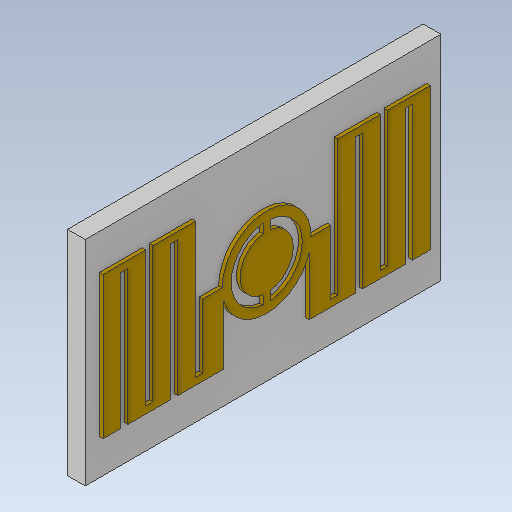
# Autodesk Inventor part: MEMS
Saved by Autodesk Inventor 2020 (Build 240168000, 168)
## iProperties
Created: 2018-12-01
Part Number: MEMS
Material: Generic
Document SubType Name: Modeling
Designer: Ralf
Density: 1 g/cm^3
Appearance: Default
Author: Ralf
Autodesk Inventor part; units mm, degrees
ref_plane "YZ Plane" through (0, 0, 0) normal (1, 0, 0) x (0, 1, 0)
ref_plane "XZ Plane" through (0, 0, 0) normal (0, 1, 0) x (-1, 0, 0)
ref_plane "XY Plane" through (0, 0, 0) normal (0, 0, 1) x (1, 0, 0)
sketch "Sketch1" plane through (0, 0, 0) normal (1, 0, 0) x (0, 1, 0)
  line L0 (-3, 5) -> (3, 5)
  line L1 (3, 5) -> (3, -5)
  line L2 (3, -5) -> (-3, -5)
  line L3 (-3, -5) -> (-3, 5)
  point P0 (0, 0)
  dimension "d0" = 6
  dimension "d1" = 10
  dimension "d2" = 3
  dimension "d3" = 5
  constraints: 8 end point, 2 parallel, 1 horizontal, 1 perpendicular
  measures "d0" distance of L0.start L0.end
  measures "d1" distance of L0.end L1.end
  measures "d2" distance from line of point (0, 0) L3
  measures "d3" distance from line of point (0, 0) L2
extrude "Extrusion1" add sketch "Sketch1" along normal blind 0.5
sketch "Sketch2" plane through (0.5, 0, 0) normal (1, 0, 0) x (0, 0, -1)
  circle A0 centre (0, 0) radius 0.75
  circle A1 centre (0, 0) radius 1
  circle A2 centre (0, 0) radius 1.25
  line L0 (-2.5, -2) -> (-2, -2)
  line L1 (-2, -2) -> (-2, 2)
  line L2 (-2, 2) -> (-2.5, 2)
  line L3 (-2.5, 2) -> (-2.5, -2)
  line L4 (-5, -3) -> (5, -3) projected
  line L5 (-3.2, -2) -> (-2.7, -2)
  line L6 (-2.7, -2) -> (-2.7, 2)
  line L7 (-2.7, 2) -> (-3.2, 2)
  line L8 (-3.2, 2) -> (-3.2, -2)
  line L9 (-3.9, -2) -> (-3.4, -2)
  line L10 (-3.4, -2) -> (-3.4, 2)
  line L11 (-3.4, 2) -> (-3.9, 2)
  line L12 (-3.9, 2) -> (-3.9, -2)
  line L13 (-4.6, -2) -> (-4.1, -2)
  line L14 (-4.1, -2) -> (-4.1, 2)
  line L15 (-4.1, 2) -> (-4.6, 2)
  line L16 (-4.6, 2) -> (-4.6, -2)
  line L17 (-0.1, -1.1173) -> (0.1, -1.1173)
  line L18 (0.1, -1.1173) -> (0.1, 1.1584)
  line L19 (0.1, 1.1584) -> (-0.1, 1.1584)
  line L20 (-0.1, 1.1584) -> (-0.1, -1.1173)
  line L21 (-1.8, -2) -> (-1.2, -2)
  line L22 (-1.2, -2) -> (-1.2, 0)
  line L23 (-1.2, 0) -> (-1.8, 0)
  line L24 (-1.8, 0) -> (-1.8, -2)
  line L25 (-1.8, -2) -> (-2, -2)
  line L26 (-2, -2) -> (-2, -1.8)
  line L27 (-2, -1.8) -> (-1.8, -1.8)
  line L28 (-1.8, -1.8) -> (-1.8, -2)
  line L29 (-2.5, 2) -> (-2.7, 2)
  line L30 (-2.7, 2) -> (-2.7, 1.8)
  line L31 (-2.7, 1.8) -> (-2.5, 1.8)
  line L32 (-2.5, 1.8) -> (-2.5, 2)
  line L33 (-3.2, -2) -> (-3.4, -2)
  line L34 (-3.4, -2) -> (-3.4, -1.8)
  line L35 (-3.4, -1.8) -> (-3.2, -1.8)
  line L36 (-3.2, -1.8) -> (-3.2, -2)
  line L37 (-3.9, 2) -> (-4.1, 2)
  line L38 (-4.1, 2) -> (-4.1, 1.8)
  line L39 (-4.1, 1.8) -> (-3.9, 1.8)
  line L40 (-3.9, 1.8) -> (-3.9, 2)
  line L41 (0, -3) -> (0, -2)
  circle A3 centre (0, 0) radius 0.75
  circle A4 centre (0, 0) radius 1
  circle A5 centre (0, 0) radius 1.25
  line L42 (2.5, -2) -> (2, -2)
  line L43 (2, -2) -> (2, 2)
  line L44 (2, 2) -> (2.5, 2)
  line L45 (2.5, 2) -> (2.5, -2)
  line L46 (3.2, -2) -> (2.7, -2)
  line L47 (2.7, -2) -> (2.7, 2)
  line L48 (2.7, 2) -> (3.2, 2)
  line L49 (3.2, 2) -> (3.2, -2)
  line L50 (3.9, -2) -> (3.4, -2)
  line L51 (3.4, -2) -> (3.4, 2)
  line L52 (3.4, 2) -> (3.9, 2)
  line L53 (3.9, 2) -> (3.9, -2)
  line L54 (4.6, -2) -> (4.1, -2)
  line L55 (4.1, -2) -> (4.1, 2)
  line L56 (4.1, 2) -> (4.6, 2)
  line L57 (4.6, 2) -> (4.6, -2)
  line L58 (0.1, -1.1173) -> (-0.1, -1.1173)
  line L59 (-0.1, -1.1173) -> (-0.1, 1.1584)
  line L60 (-0.1, 1.1584) -> (0.1, 1.1584)
  line L61 (0.1, 1.1584) -> (0.1, -1.1173)
  line L62 (1.8, -2) -> (1.2, -2)
  line L63 (1.2, -2) -> (1.2, 0)
  line L64 (1.2, 0) -> (1.8, 0)
  line L65 (1.8, 0) -> (1.8, -2)
  line L66 (1.8, -2) -> (2, -2)
  line L67 (2, -2) -> (2, -1.8)
  line L68 (2, -1.8) -> (1.8, -1.8)
  line L69 (1.8, -1.8) -> (1.8, -2)
  line L70 (2.5, 2) -> (2.7, 2)
  line L71 (2.7, 2) -> (2.7, 1.8)
  line L72 (2.7, 1.8) -> (2.5, 1.8)
  line L73 (2.5, 1.8) -> (2.5, 2)
  line L74 (3.2, -2) -> (3.4, -2)
  line L75 (3.4, -2) -> (3.4, -1.8)
  line L76 (3.4, -1.8) -> (3.2, -1.8)
  line L77 (3.2, -1.8) -> (3.2, -2)
  line L78 (3.9, 2) -> (4.1, 2)
  line L79 (4.1, 2) -> (4.1, 1.8)
  line L80 (4.1, 1.8) -> (3.9, 1.8)
  line L81 (3.9, 1.8) -> (3.9, 2)
  dimension "d6" = 1.5
  dimension "d7" = 2
  dimension "d8" = 2.5
  dimension "d9" = 0.5
  dimension "d10" = 4
  dimension "d11" = 1
  dimension "d14" = 0.7
  dimension "d19" = 0.2
  dimension "d20" = 0.1
  dimension "d21" = 2
  dimension "d22" = 0.6
  dimension "d23" = 2
  dimension "d24" = 0.2
  dimension "d25" = 0.2
  dimension "d26" = 0.2
  dimension "d27" = 0.2
  dimension "d28" = 0.2
  constraints: 162 end point, 36 symmetric about line, 14 parallel, 8 horizontal, 8 point on line, 7 perpendicular, 6 centre point, 6 coincident, 1 collinear, 1 midpoint, 1 vertical, 26 other
  measures "d6" diameter of A0
  measures "d7" diameter of A1
  measures "d8" diameter of A2
  measures "d9" distance of L2.end L1.end
  measures "d10" distance of L1.end L0.end
  measures "d11" distance between parallel lines of L0 L4
  measures "d14" distance of L0.start L5.start
  measures "d19" distance of L18.end L19.end
  measures "d20" distance from line of point (0, 0) L18
  measures "d21" distance from line of point (0, 0) L1
  measures "d22" distance of L23.end L22.end
  measures "d23" distance of L22.end L21.end
  measures "d24" distance between parallel lines of L24 L1
  measures "d25" distance of L25.end L26.end
  measures "d26" distance of L30.end L29.end
  measures "d27" distance of L33.end L34.end
  measures "d28" distance of L38.end L37.end
extrude "Extrusion2" add sketch "Sketch2" along normal blind 0.1 contours A0 L18 | L18 A0 L20 | A0 L20 A1 L18 | L18 A1 L20 A0 | L20 A0 | A1 L20 L19 L18 | L18 L17 L20 A1 | L64 L63 A2 L22 L23 | L64 L65 L62 L63 A2 | A2 L63 L64 | L23 L22 A2 | A2 L22 L21 L24 L23 | L68 L43 L66 L65 | L24 L25 L1 L27 | L43 L44 L45 L42 | L1 L0 L3 L2 | L70 L47 L72 L45 | L3 L31 L6 L29 | L48 L49 L46 L47 | L6 L5 L8 L7 | L76 L51 L74 L49 | L8 L33 L10 L35 | L51 L52 L53 L50 | L10 L9 L12 L11 | L78 L55 L80 L53 | L12 L39 L14 L37 | L56 L57 L54 L55 | L14 L13 L16 L15
body "Solid1"
